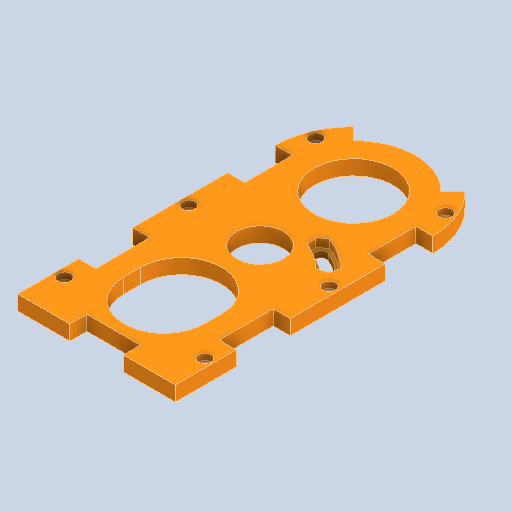
# Autodesk Inventor part: Primer segmento - inferior v1.2
Saved by Autodesk Inventor 2026 (Build 300175050, 175E)
## iProperties
Created: 2025-07-19
Part Number: Primer segmento - inferior v1.2
Material: Plastico PETG
Document SubType Name: Modeling
Designer: bello
Density: 1.27 g/cm^3
Appearance: Naranja
Author: bello
Autodesk Inventor part; units mm, degrees
ref_plane "YZ Plane" through (0, 0, 0) normal (1, 0, 0) x (0, 1, 0)
ref_plane "XZ Plane" through (0, 0, 0) normal (0, 1, 0) x (-1, 0, 0)
ref_plane "XY Plane" through (0, 0, 0) normal (0, 0, 1) x (1, 0, 0)
sketch "Boceto1" plane through (0, 0, 0) normal (0, 1, 0) x (-1, 0, 0)
  line L0 (0, 0) -> (-24.6, 0)
  line L1 (0, 0) -> (0, -29)
  line L2 (0, -29) -> (-8, -29)
  line L3 (-8, -29) -> (-8, -54)
  line L4 (-8, -54) -> (0, -54)
  line L5 (0, -54) -> (0, -99)
  line L6 (0, -99) -> (-8, -99)
  line L7 (-8, -99) -> (-8, -121)
  line L8 (-8, -121) -> (0, -121)
  line L9 (-24.6, 0) -> (-24.6, -8)
  line L10 (-24.6, -8) -> (-49.4, -8)
  line L11 (-37, 21.7087) -> (-37, -150)
  arc A0 (-57.5061, -141.5061) -> (-16.4939, -141.5061) centre (-37, -121) ccw
  line L12 (-37, -121) -> (-16.4939, -141.5061)
  line L13 (-16.4939, -141.5061) -> (-10.837, -147.163)
  line L14 (-74, 0) -> (-49.4, 0)
  line L15 (-74, 0) -> (-74, -29)
  line L16 (-74, -29) -> (-66, -29)
  line L17 (-66, -29) -> (-66, -54)
  line L18 (-66, -54) -> (-74, -54)
  line L19 (-74, -54) -> (-74, -99)
  line L20 (-74, -99) -> (-66, -99)
  line L21 (-66, -99) -> (-66, -121)
  line L22 (-66, -121) -> (-74, -121)
  line L23 (-49.4, 0) -> (-49.4, -8)
  line L24 (-37, -121) -> (-57.5061, -141.5061)
  line L25 (-57.5061, -141.5061) -> (-63.163, -147.163)
  arc A1 (-74, -121) -> (-63.163, -147.163) centre (-37, -121) ccw
  arc A2 (-10.837, -147.163) -> (0, -121) centre (-37, -121) ccw
  dimension "d139" = 24.6
  dimension "d140" = 29
  dimension "d141" = 25
  dimension "d142" = 8
  dimension "d143" = 45
  dimension "d144" = 22
  dimension "d145" = 8
  dimension "d146" = 24.8
  dimension "d148" = 45
  constraints: 52 end point, 12 symmetric about line, 8 point on line, 7 point on circle, 5 perpendicular, 3 centre point, 3 horizontal, 3 vertical, 1 coincident, 1 other
  measures "d139" distance of L0.start L0.end
  measures "d140" distance of L0.start L1.end
  measures "d141" distance of L2.end L3.end
  measures "d142" distance of L1.end L2.end
  measures "d143" distance of L4.end L5.end
  measures "d144" distance of L6.end L7.end
  measures "d145" distance of L0.end L9.end
  measures "d146" distance of L9.end L10.end
  measures "d148" angle of L8 L13
extrude "Extrusión1" add sketch "Boceto1" along normal blind 7
sketch "Boceto2" plane through (0, 7, 0) normal (0, 1, 0) x (1, 0, 0)
  arc A0 (18, 32) -> (56, 32) centre (37, 32) ccw
  arc A1 (56, 40) -> (18, 40) centre (37, 40) ccw
  line L0 (18, 40) -> (18, 32)
  line L1 (56, 32) -> (56, 40)
  circle A2 centre (37, 77) radius 11.1
  circle A3 centre (37, 121) radius 18.6
  line L2 (37, -3.2334) -> (37, 158.5758)
  point P0 (0, 0)
  dimension "d18" = 19
  dimension "d23" = 22.2
  dimension "d25" = 37.2
  dimension "d149" = 44
  dimension "d150" = 37
  dimension "d151" = 8
  constraints: 6 end point, 4 centre point, 4 point on circle, 3 vertical, 1 parallel
  measures "d18" radius of A1
  measures "d23" diameter of A2
  measures "d25" diameter of A3
  measures "d149" distance of A2.centre A3.centre
  measures "d150" distance of A1.centre A2.centre
  measures "d151" distance of A0.centre A1.centre
extrude "Extrusión2" cut sketch "Boceto2" against normal blind 7
sketch "Boceto3" plane through (0, 7, 0) normal (0, 1, 0) x (1, 0, 0)
  line L0 (37, -12.6618) -> (37, 178.5268)
  circle A0 centre (4, 18) radius 2.05
  circle A1 centre (4, 76.5) radius 2.05
  circle A2 centre (37, 121) radius 18.6 projected
  circle A3 centre (37, 121) radius 33
  circle A4 centre (6.512, 133.6286) radius 2.05
  line L1 (8, 29) -> (0, 29) projected
  line L2 (0, 29) -> (0, 0) projected
  line L3 (0, 99) -> (0, 54) projected
  line L4 (8, 99) -> (0, 99) projected
  line L5 (6.512, 133.6286) -> (37, 121)
  line L6 (24.8695, 121) -> (50.3921, 121)
  circle A5 centre (70, 18) radius 2.05
  circle A6 centre (70, 76.5) radius 2.05
  circle A7 centre (67.488, 133.6286) radius 2.05
  line L7 (67.488, 133.6286) -> (37, 121)
  dimension "d157" = 66
  dimension "d152" = 11
  dimension "d153" = 4
  dimension "d154" = 4.1
  dimension "d155" = 4
  dimension "d156" = 22.5
  dimension "d158" = 22.5
  constraints: 8 end point, 6 centre point, 3 symmetric about line, 2 equal radius, 1 coincident, 1 horizontal, 1 vertical, 6 other
  measures "d152" distance from line of A0.centre L1
  measures "d153" distance from line of L2 A0.centre
  measures "d154" diameter of A0
  measures "d155" distance from line of L3 A1.centre
  measures "d156" distance from line of L4 A1.centre
  measures "d158" angle of L6 L5
extrude "Extrusión3" cut sketch "Boceto3" against normal through all contours A4 A3 | A3 L5 A4 | A3 A4 L5 | A7 L7 A3 | A3 A7 | L7 A7 A3 | A0 | A1 | A5 | A6
sketch "Boceto12" plane through (0, 7, 0) normal (0, 1, 0) x (1, 0, 0)
  circle A0 centre (37, 77) radius 11.1 projected
  circle A1 centre (37, 121) radius 18.6 projected
  arc A2 (60.7956, 85.0881) -> (51.3765, 91.3074) centre (38.4503, 61.4886) ccw
  line L0 (38.4503, 61.4886) -> (60.7956, 85.0881)
  line L1 (38.4503, 61.4886) -> (51.3765, 91.3074)
  line L2 (51.3765, 91.3074) -> (52.4106, 93.693)
  line L3 (60.7956, 85.0881) -> (62.5832, 86.9761)
  line L4 (38.4503, 61.4886) -> (51.3765, 91.3074)
  line L5 (50.3411, 88.9225) -> (50.3424, 88.9219)
  line L6 (59.009, 83.1992) -> (59.008, 83.2002)
  circle A3 centre (51.3765, 91.3074) radius 2.6
  circle A4 centre (60.7956, 85.0881) radius 2.6
  circle A5 centre (38.4503, 61.4886) radius 29.9
  circle A6 centre (38.4503, 61.4886) radius 35.1
  point P0 (0, 0)
  point P1 (59.009, 83.1992)
  dimension "d101" = 0
  dimension "d102" = 20
  dimension "d91" = 65
  dimension "d173" = 5.2
  dimension "d174" = 5.2
  constraints: 6 coincident, 4 end point, 3 centre point, 3 point on circle, 24 other
  measures "d91" diameter of A2
  measures "d173" diameter of A3
  measures "d174" diameter of A4
extrude "Extrusión10" cut sketch "Boceto12" against normal through all contours A3 L2 L1 | L1 A2 A3 | A3 A2 A4 A5 | L2 A3 A2 | A6 A4 A2 A3 | A4 A2 L0 | L0 L3 A4 | L3 A2 A4
sketch "Boceto13" plane through (0, 7, 0) normal (0, 1, 0) x (1, 0, 0)
  line L0 (47.0857, 93.1674) -> (50.8419, 95.9533)
  line L1 (50.8419, 95.9533) -> (52.9888, 95.0227)
  line L2 (49.7657, 87.5915) -> (47.6203, 88.5215)
  line L3 (47.6203, 88.5215) -> (47.0857, 93.1674)
  line L4 (59.7114, 80.539) -> (57.9998, 82.1579)
  line L5 (63.5861, 88.0233) -> (65.2773, 86.4238)
  line L6 (65.2773, 86.4238) -> (64.1931, 81.8747)
  line L7 (64.1931, 81.8747) -> (59.7114, 80.539)
  circle A0 centre (38.4503, 61.4886) radius 28.45
  circle A1 centre (38.4503, 61.4886) radius 36.55
  point P0 (0, 0)
  point P1 (51.3765, 91.3074)
  point P2 (60.7956, 85.0881)
  point P3 (60.7956, 85.0881)
  point P4 (51.3765, 91.3074)
  point P5 (51.3765, 91.3074)
  point P6 (51.3765, 91.3074)
  point P7 (60.7956, 85.0881)
  point P8 (65.2562, 86.3351)
  point P9 (50.7698, 95.8998)
  dimension "d172" = 8.1
  constraints: 16 end point, 5 coincident, 4 point on circle, 2 centre point, 12 other
  measures "d172" distance between parallel lines of L5 L4
extrude "Extrusión11" cut sketch "Boceto13" against normal blind 4 contours L0 A1 L6 L7 L4 A0 L2 L3 picked at (62.116, 83.8351)
sketch "Boceto15" plane through (0, 7, 0) normal (0, 1, 0) x (1, 0, 0)
  circle A0 centre (4.0687, 18) radius 3
  circle A1 centre (4, 76.5) radius 2.05 projected
  circle A2 centre (4, 76.5) radius 3
  circle A3 centre (6.512, 133.6286) radius 2.05 projected
  circle A4 centre (6.512, 133.6286) radius 3
  circle A5 centre (67.488, 133.6286) radius 2.05 projected
  circle A6 centre (67.488, 133.6286) radius 3
  circle A7 centre (70, 76.5) radius 2.05 projected
  circle A8 centre (70, 76.5) radius 3
  circle A9 centre (70, 18) radius 2.05 projected
  circle A10 centre (70, 18) radius 3
  point P0 (0, 0)
  dimension "d159" = 6
  dimension "d160" = 6
  dimension "d161" = 6
  dimension "d162" = 6
  dimension "d163" = 6
  dimension "d164" = 6
  constraints: 6 centre point, 5 coincident
  measures "d159" diameter of A0
  measures "d160" diameter of A2
  measures "d161" diameter of A4
  measures "d162" diameter of A6
  measures "d163" diameter of A8
  measures "d164" diameter of A10
extrude "Extrusión12" cut sketch "Boceto15" against normal blind 3 contours A0 | A1 | A2 | A3 | A4 | A5 | A6 | A7 | A8 | A9 | A10
sketch "Boceto16" plane through (0, 7, 0) normal (0, 1, 0) x (1, 0, 0)
  line L0 (0, 29) -> (0, 0) projected
  line L1 (0, 29) -> (8, 29)
  line L2 (8, 29) -> (8, 28.8)
  line L3 (8, 28.8) -> (0, 28.8)
  line L4 (0, 28.8) -> (0, 29)
  line L5 (0, 54) -> (8, 54) projected
  line L6 (0, 54) -> (8, 54)
  line L7 (8, 54) -> (8, 54.2)
  line L8 (8, 54.2) -> (0, 54.2)
  line L9 (0, 54.2) -> (0, 54)
  line L10 (8, 99) -> (0, 99) projected
  line L11 (0, 99) -> (8, 99)
  line L12 (8, 99) -> (8, 98.8)
  line L13 (8, 98.8) -> (0, 98.8)
  line L14 (0, 98.8) -> (0, 99)
  line L15 (8, 121) -> (8, 99) projected
  line L16 (8, 121) -> (0, 121)
  line L17 (0, 121) -> (0, 121.2)
  line L18 (0, 121.2) -> (8, 121.2)
  line L19 (8, 121.2) -> (8, 121)
  line L20 (16.4939, 141.5061) -> (10.837, 147.163) projected
  line L21 (16.4939, 141.5061) -> (16.3525, 141.3647)
  line L22 (16.3525, 141.3647) -> (10.6956, 147.0215)
  line L23 (10.6956, 147.0215) -> (10.837, 147.163)
  line L24 (24.6, 0) -> (24.6, 8) projected
  line L25 (0, 0) -> (24.6, 0)
  line L26 (24.6, 0) -> (24.6, 0.2)
  line L27 (24.6, 0.2) -> (0, 0.2)
  line L28 (0, 0.2) -> (0, 0)
  line L29 (24.6, 8) -> (49.4, 8) projected
  line L30 (24.6, 8) -> (24.4, 8)
  line L31 (24.4, 8) -> (24.4, 0)
  line L32 (24.4, 0) -> (24.6, 0)
  line L33 (24.6, 0) -> (24.6, 8)
  line L34 (37, -18.4316) -> (37, 165.7514)
  line L35 (74, 29) -> (74, 0)
  line L36 (74, 29) -> (66, 29)
  line L37 (66, 29) -> (66, 28.8)
  line L38 (66, 28.8) -> (74, 28.8)
  line L39 (74, 28.8) -> (74, 29)
  line L40 (74, 54) -> (66, 54)
  line L41 (74, 54) -> (66, 54)
  line L42 (66, 54) -> (66, 54.2)
  line L43 (66, 54.2) -> (74, 54.2)
  line L44 (74, 54.2) -> (74, 54)
  line L45 (66, 99) -> (74, 99)
  line L46 (74, 99) -> (66, 99)
  line L47 (66, 99) -> (66, 98.8)
  line L48 (66, 98.8) -> (74, 98.8)
  line L49 (74, 98.8) -> (74, 99)
  line L50 (66, 121) -> (66, 99)
  line L51 (66, 121) -> (74, 121)
  line L52 (74, 121) -> (74, 121.2)
  line L53 (74, 121.2) -> (66, 121.2)
  line L54 (66, 121.2) -> (66, 121)
  line L55 (57.5061, 141.5061) -> (63.163, 147.163)
  line L56 (57.5061, 141.5061) -> (57.6475, 141.3647)
  line L57 (57.6475, 141.3647) -> (63.3044, 147.0215)
  line L58 (63.3044, 147.0215) -> (63.163, 147.163)
  line L59 (49.4, 0) -> (49.4, 8)
  line L60 (74, 0) -> (49.4, 0)
  line L61 (49.4, 0) -> (49.4, 0.2)
  line L62 (49.4, 0.2) -> (74, 0.2)
  line L63 (74, 0.2) -> (74, 0)
  line L64 (49.4, 8) -> (49.6, 8)
  line L65 (49.6, 8) -> (49.6, 0)
  line L66 (49.6, 0) -> (49.4, 0)
  line L67 (49.4, 0) -> (49.4, 8)
  line L68 (24.4, 8) -> (49.6, 8)
  line L69 (49.6, 8) -> (49.6, 8.2)
  line L70 (49.6, 8.2) -> (24.4, 8.2)
  line L71 (24.4, 8.2) -> (24.4, 8)
  point P0 (24.4, 0.2)
  point P1 (0, 0.2)
  point P2 (49.6, 0.2)
  dimension "d166" = 8
  dimension "d167" = 0.2
  dimension "d168" = 0.2
  dimension "d169" = 0.2
  constraints: 130 end point, 30 symmetric about line, 14 parallel, 10 point on line, 9 perpendicular, 7 horizontal, 5 equal length, 1 vertical
  measures "d166" distance of L21.end L22.end
  measures "d167" distance of L1.end L2.end
  measures "d168" distance between parallel lines of L25 L27
  measures "d169" distance of L68.end L69.end
extrude "Extrusión13" cut sketch "Boceto16" against normal through all
